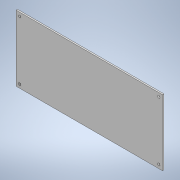
# Autodesk Inventor part: 20220523_知能ロボット2階部分
Saved by Autodesk Inventor 2020 (Build 240168000, 168)
## iProperties
Created: 2022-05-22
Part Number: 20220523_知能ロボット2階部分
Material: 一般
Document SubType Name: Modeling
Designer: Naggy
Density: 1 g/cm^3
Appearance: 既定
Author: Naggy
Autodesk Inventor part; units mm, degrees
ref_plane "YZ Plane" through (0, 0, 0) normal (1, 0, 0) x (0, 1, 0)
ref_plane "XZ Plane" through (0, 0, 0) normal (0, 1, 0) x (-1, 0, 0)
ref_plane "XY Plane" through (0, 0, 0) normal (0, 0, 1) x (1, 0, 0)
sketch "スケッチ1" plane through (0, 0, 0) normal (0, 0, 1) x (1, 0, 0)
  line L0 (-100, -45) -> (100, -45)
  line L1 (100, -45) -> (100, 45)
  line L2 (100, 45) -> (-100, 45)
  line L3 (-100, 45) -> (-100, -45)
  line L4 (-100, -45) -> (100, 45) construction
  line L5 (100, -45) -> (-100, 45) construction
  point P0 (0, 0)
  dimension "d0" = 90
  dimension "d1" = 200
  constraints: 12 end point, 2 midpoint, 2 parallel, 1 horizontal, 1 perpendicular
  measures "d0" distance between parallel lines of L0 L2
  measures "d1" distance between parallel lines of L1 L3
extrude "押し出し1" add sketch "スケッチ1" along normal blind 2
sketch "スケッチ2" plane through (0, 0, 2) normal (0, 0, 1) x (1, 0, 0)
  line L0 (100, 45) -> (-100, 45) projected
  line L1 (-100, 45) -> (-100, -45) projected
  line L2 (100, -45) -> (100, 45) projected
  line L3 (-100, -45) -> (100, -45) projected
  point P0 (0, 0)
  point P1 (-95, -40)
  point P2 (95, -40)
  point P3 (-95, 40)
  point P4 (95, 40)
  dimension "d4" = 5
  dimension "d5" = 5
  dimension "d6" = 5
  dimension "d7" = 5
  dimension "d8" = 5
  dimension "d9" = 5
  dimension "d10" = 5
  dimension "d11" = 5
  measures "d4" distance from line of point (-95, 40) L0
  measures "d5" distance from line of point (-95, 40) L1
  measures "d6" distance from line of L0 point (95, 40)
  measures "d7" distance from line of point (95, 40) L2
  measures "d8" distance from line of point (-95, -40) L1
  measures "d9" distance from line of point (-95, -40) L3
  measures "d10" distance from line of point (95, -40) L3
  measures "d11" distance from line of point (95, -40) L2
hole "穴1" at (-95, -40, 2) at (95, -40, 2) at (-95, 40, 2) at (95, 40, 2) direction (0, 0, -1) diameter 3.4 end through all clearance for "Flat Head Machine Screw" size "M3" standard "Ansi Metric M Profile"
